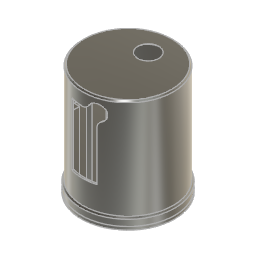
meshtastic-heltec-holder v7 (Autodesk Fusion 360 design; units mm, degrees)
Autodesk Fusion 360 part; units mm, degrees
note: some values were not read from the file. Set by a fixed rule: which sketch regions a step uses.
sketch "boden" plane through (0, 0, 0) normal (0, 0, 1) x (1, 0, 0)
  circle A0 centre (0, 0) radius 30
  line L0 (-11, -23) -> (11, -23)
  line L1 (11, -23) -> (11, -15)
  line L2 (11, -15) -> (-11, -15)
  line L3 (-11, -15) -> (-11, -23)
  line L4 (-11, -23) -> (-8, -23)
  line L5 (-8, -23) -> (-8, -25)
  line L6 (-8, -25) -> (-11, -25)
  line L7 (-11, -25) -> (-11, -23)
  line L8 (11, -23) -> (8, -23)
  line L9 (8, -23) -> (8, -25)
  line L10 (8, -25) -> (11, -25)
  line L11 (11, -25) -> (11, -23)
  line L12 (-11, -15) -> (-8, -15)
  line L13 (-8, -15) -> (-8, -13)
  line L14 (-8, -13) -> (-11, -13)
  line L15 (-11, -13) -> (-11, -15)
  line L16 (11, -15) -> (8, -15)
  line L17 (8, -15) -> (8, -13)
  line L18 (8, -13) -> (11, -13)
  line L19 (11, -13) -> (11, -15)
  line L20 (11, -13) -> (13, -13)
  line L21 (13, -13) -> (13, -25)
  line L22 (13, -25) -> (11, -25)
  line L23 (11, -25) -> (11, -13)
  line L24 (-11, -25) -> (-13, -25)
  line L25 (-13, -25) -> (-13, -13)
  line L26 (-13, -13) -> (-11, -13)
  line L27 (-11, -13) -> (-11, -25)
  line L28 (8, -15) -> (-8, -15)
  line L29 (-8, -15) -> (-8, -6)
  line L30 (-8, -6) -> (8, -6)
  line L31 (8, -6) -> (8, -15)
  line L32 (-13, -13) -> (-11, -13)
  line L33 (-11, -13) -> (-11, -4)
  line L34 (-11, -4) -> (-13, -4)
  line L35 (-13, -4) -> (-13, -13)
  line L36 (13, -4) -> (13, -6)
  line L37 (13, -6) -> (-11, -6)
  line L38 (-11, -6) -> (-11, -4)
  line L39 (11, -13) -> (13, -13)
  line L40 (13, -13) -> (13, -6)
  line L41 (13, -6) -> (11, -6)
  line L42 (11, -6) -> (11, -13)
  line L43 (13, -4) -> (3, -4)
  line L44 (3, -4) -> (3, -6)
  line L45 (3, -6) -> (13, -6)
  line L46 (13, -6) -> (13, -4)
  line L47 (-11, -4) -> (-3, -4)
  line L48 (-3, -4) -> (-3, -6)
  line L49 (-3, -6) -> (-11, -6)
  line L50 (-11, -6) -> (-11, -4)
  line L51 (-26.5, -4) -> (26.5, -4)
  line L52 (26.5, -4) -> (26.5, 2)
  line L53 (26.5, 2) -> (-26.5, 2)
  line L54 (-26.5, 2) -> (-26.5, -4)
  line L55 (-13, -5) -> (-13, -4)
  line L56 (-13, -4) -> (-27.5, -4)
  line L57 (-27.5, -4) -> (-27.5, -5)
  line L58 (-27.5, -5) -> (-13, -5)
  line L59 (-13, -5) -> (-13, -4)
  line L60 (-26.5, -4) -> (-27.5, -4)
  line L61 (-27.5, -4) -> (-27.5, 3)
  line L62 (-27.5, 3) -> (-26.5, 3)
  line L63 (-26.5, 3) -> (-26.5, -4)
  line L64 (-26.5, 3) -> (27.5, 3)
  line L65 (27.5, 3) -> (27.5, 2)
  line L66 (27.5, 2) -> (-26.5, 2)
  line L67 (-26.5, 2) -> (-26.5, 3)
  line L68 (27.5, 2) -> (26.5, 2)
  line L69 (26.5, 2) -> (26.5, -5)
  line L70 (26.5, -5) -> (27.5, -5)
  line L71 (27.5, -5) -> (27.5, 2)
  line L72 (26.5, -5) -> (13, -5)
  line L73 (13, -5) -> (13, -4)
  line L74 (13, -4) -> (26.5, -4)
  line L75 (26.5, -4) -> (26.5, -5)
  line L76 (2, 2) -> (-2, 2)
  line L77 (-2, 2) -> (-2, 3)
  line L78 (-2, 3) -> (2, 3)
  line L79 (2, 3) -> (2, 2)
  line L80 (10, 3) -> (-10, 3)
  line L81 (-10, 3) -> (-10, 17)
  line L82 (-10, 17) -> (10, 17)
  line L83 (10, 17) -> (10, 3)
  line L84 (8, 17) -> (-8, 17)
  line L85 (-8, 17) -> (-8, 5)
  line L86 (-8, 5) -> (8, 5)
  line L87 (8, 5) -> (8, 17)
  line L88 (2, 3) -> (-2, 3)
  line L89 (-2, 5) -> (2, 5)
  line L90 (1, 3) -> (-1, 3)
  line L91 (-1, 3) -> (-1, 5)
  line L92 (-1, 5) -> (1, 5)
  line L93 (1, 5) -> (1, 3)
  line L94 (1, 5) -> (-1, 5)
  line L95 (-1, 5) -> (-1, 13)
  line L96 (-1, 13) -> (1, 13)
  line L97 (1, 13) -> (1, 5)
  circle A1 centre (0, 13) radius 3.1
  circle A2 centre (0, 0) radius 28
  circle A3 centre (0, 0) radius 29
  line L98 (-27.8388, 3) -> (-27.5, 3)
  line L99 (-25.5, 3) -> (-25.5, 7.5)
  line L100 (-25.5, 7.5) -> (-26.9768, 7.5)
  line L101 (27.5, 3) -> (27.8388, 3)
  line L102 (0, 0) -> (0, 40) construction
  line L103 (25.5, 3) -> (25.5, 7.5)
  line L104 (25.5, 7.5) -> (26.9768, 7.5)
  line L105 (-5, 5) -> (5, 5)
  line L106 (5, 5) -> (5, 2)
  line L107 (5, 2) -> (-5, 2)
  line L108 (-5, 2) -> (-5, 5)
  line L109 (27.5, -5) -> (27.55, -5)
  line L110 (-27.5, -4) -> (-27.7128, -4)
  line L111 (-8, -25) -> (-8, -26.8328)
  line L112 (8, -25) -> (8, -26.8328)
  circle A4 centre (0, 13) radius 6.75
  dimension "d1" = 60
  dimension "d4" = 22
  dimension "d5" = 8
  dimension "d6" = 11
  dimension "d7" = 15
  dimension "d8" = 53
  dimension "d9" = 6
  dimension "d10" = 1
  dimension "d11" = 26.5
  dimension "d18" = 6.2
  dimension "d23" = 58
  dimension "d24" = 40
  dimension "d37" = 13.5
  constraint coincident A0.centre A2.centre
  constraint horizontal L0
  constraint vertical L1
  constraint horizontal L2
  constraint vertical L3
  constraint horizontal L4
  constraint vertical L5
  constraint horizontal L6
  constraint vertical L7
  constraint horizontal L8
  constraint vertical L9
  constraint horizontal L10
  constraint vertical L11
  constraint horizontal L12
  constraint vertical L13
  constraint horizontal L14
  constraint vertical L15
  constraint horizontal L16
  constraint vertical L17
  constraint horizontal L18
  constraint vertical L19
  constraint horizontal L20
  constraint vertical L21
  constraint horizontal L22
  constraint vertical L23
  constraint horizontal L24
  constraint vertical L25
  constraint horizontal L26
  constraint vertical L27
  constraint horizontal L28
  constraint vertical L29
  constraint horizontal L30
  constraint vertical L31
  constraint horizontal L32
  constraint vertical L33
  constraint horizontal L34
  constraint vertical L35
  constraint vertical L36
  constraint horizontal L37
  constraint vertical L38
  constraint horizontal L39
  constraint vertical L40
  constraint horizontal L41
  constraint vertical L42
  constraint horizontal L43
  constraint vertical L44
  constraint horizontal L45
  constraint vertical L46
  constraint coincident L30 L44.end
  constraint coincident L37 L44.end
  constraint horizontal L47
  constraint vertical L48
  constraint horizontal L49
  constraint vertical L50
  constraint coincident L30 L48.end
  constraint horizontal L51
  constraint vertical L52
  constraint horizontal L53
  constraint vertical L54
  constraint vertical L55
  constraint horizontal L56
  constraint vertical L57
  constraint horizontal L58
  constraint vertical L59
  constraint horizontal L60
  constraint vertical L61
  constraint horizontal L62
  constraint vertical L63
  constraint horizontal L64
  constraint vertical L65
  constraint horizontal L66
  constraint vertical L67
  constraint horizontal L68
  constraint vertical L69
  constraint horizontal L70
  constraint vertical L71
  constraint horizontal L72
  constraint vertical L73
  constraint horizontal L74
  constraint vertical L75
  constraint horizontal L76
  constraint vertical L77
  constraint horizontal L78
  constraint vertical L79
  constraint coincident L64 L77.end
  constraint horizontal L80
  constraint vertical L81
  constraint horizontal L82
  constraint vertical L83
  constraint coincident L64 L80.start
  constraint horizontal L84
  constraint vertical L85
  constraint horizontal L86
  constraint vertical L87
  constraint coincident L82 L84.start
  constraint horizontal L88
  constraint horizontal L89
  constraint coincident L86 L89.start
  constraint horizontal L90
  constraint vertical L91
  constraint horizontal L92
  constraint vertical L93
  constraint coincident L89 L91.end
  constraint coincident L80 L90.start
  constraint horizontal L94
  constraint vertical L95
  constraint horizontal L96
  constraint vertical L97
  constraint midpoint L96 A1.centre
  constraint coincident A2 L98.start
  constraint perpendicular L61 L98
  constraint coincident L64 L99.start
  constraint perpendicular L64 L99
  constraint coincident A2 L100.end
  constraint perpendicular L99 L100
  constraint coincident A2 L101.end
  constraint perpendicular L65 L101
  constraint vertical L102
  constraint symmetric L99.start L102 L103.start
  constraint symmetric L99.end L102 L103.end
  constraint symmetric L100.end L102 L104.end
  constraint horizontal L105
  constraint vertical L106
  constraint horizontal L107
  constraint vertical L108
  constraint coincident L53 L106.end
  constraint coincident L86 L105.start
  constraint coincident A2 L109.end
  constraint perpendicular L71 L109
  constraint coincident A2 L110.end
  constraint perpendicular L57 L110
  constraint coincident A2 L111.end
  constraint perpendicular L6 L111
  constraint coincident A2 L112.end
  constraint perpendicular L10 L112
  constraint concentric A1 A4
  measures "d1" diameter of A0
  measures "d4" distance of L0.start L0.end
  measures "d5" distance of L0.start L2.end
  measures "d6" distance of A0.centre L1
  measures "d7" distance of A0.centre L28
  measures "d8" distance of L51.start L51.end
  measures "d9" distance of L51.start L53.end
  measures "d10" distance of L54 L57
  measures "d11" distance of A0.centre L54
  measures "d18" diameter of A1
  measures "d23" diameter of A3
  measures "d24" distance of A0.centre L102.end
  measures "d37" diameter of A4
extrude "Extrude1" add sketch "boden" against normal blind 2 contours A0 | L0 L1 L2 L3 L4 L8 L12 L16 L23 L27 L28 | L3 L7 L15 L24 L25 L26 L27 L32 A2 | L0 L4 L5 L6 L7 L27 | L0 L5 L9 A2 L111 L112 | L2 L12 L13 L14 L15 L27 L29 | L6 L24 A2 L111 | L0 L8 L9 L10 L11 L23 | L2 L13 L17 L28 L29 L30 L31 L37 L45 L49 | L14 L29 L33 L37 L49 | L26 L32 L33 L34 L35 L38 L50 L51 L55 L59 | L24 L25 A2 | L1 L11 L19 L20 L21 L22 L23 L39 A2 | L10 L22 A2 L112 | L2 L16 L17 L18 L19 L23 L31 | L25 L35 L57 L58 A2 L110 | L30 L33 L37 L38 L47 L48 L49 L50 L51 | L18 L31 L37 L42 L45 | L35 L51 L55 L56 L57 L58 L59 L60 | L34 L43 L47 L51 L52 L53 L54 L56 L63 L66 L69 L74 L76 L107 | L61 A2 L98 L110 | L20 L37 L39 L40 L41 L42 L45 | L21 L22 A2 | L30 L36 L37 L41 L43 L44 L45 L46 L51 L73 | L30 L37 L44 L48 L51 | L62 L64 A2 L98 L99 L100 | L54 L56 L60 L61 L62 L63 L67 | L21 L36 L40 L46 L70 L72 A2 L109 | L64 L81 L82 L83 L84 A2 L99 L100 L103 L104 A4 | L65 L71 A2 L101 L109 | L53 L63 L64 L66 L67 L80 L108 | L36 L46 L51 L69 L72 L73 L74 L75 | L64 A2 L101 L103 L104 | L52 L66 L68 L69 L70 L71 L75 | L53 L64 L66 L77 L80 L107 L108 | L53 L64 L65 L66 L68 L80 L106 | L53 L64 L66 L76 L77 L78 L79 L80 L88 L90 L107 | L64 L78 L80 L86 L88 L89 L91 L105 L108 | L64 L80 L81 L82 L85 L86 L108 | L53 L64 L66 L79 L80 L106 L107 | L82 L84 L85 L86 L89 L95 L105 A4 | L64 L80 L82 L83 L86 L87 L106 | L64 L78 L80 L86 L88 L89 L93 L105 L106 | L64 L78 L80 L86 L88 L89 L90 L91 L92 L93 L94 L105 | L86 L89 L92 L94 L95 L97 L105 A4 | L82 L84 L86 L87 L89 L97 L105 A4 | L82 L84 A4 | L82 L84 L95 L97 A1 A4 | L95 L97 A1 A4 | L95 L96 L97 A1 | L95 L96 L97 A1 | A3 makes body 1
extrude "Extrude2" add sketch "boden" along normal blind 48 contours L3 L7 L15 L24 L25 L26 L27 L32 A2 | L0 L4 L5 L6 L7 L27 | L2 L12 L13 L14 L15 L27 L29 | L0 L8 L9 L10 L11 L23 | L14 L29 L33 L37 L49 | L26 L32 L33 L34 L35 L38 L50 L51 L55 L59 | L24 L25 A2 | L1 L11 L19 L20 L21 L22 L23 L39 A2 | L2 L16 L17 L18 L19 L23 L31 | L30 L33 L37 L38 L47 L48 L49 L50 L51 | L18 L31 L37 L42 L45 | L20 L37 L39 L40 L41 L42 L45 | L21 L22 A2 | L30 L36 L37 L41 L43 L44 L45 L46 L51 L73 bodies 1
extrude "Extrude3" add sketch "boden" along normal blind 60 contours L35 L51 L55 L56 L57 L58 L59 L60 | L54 L56 L60 L61 L62 L63 L67 | L53 L63 L64 L66 L67 L80 L108 | L36 L46 L51 L69 L72 L73 L74 L75 | L52 L66 L68 L69 L70 L71 L75 | L53 L64 L66 L77 L80 L107 L108 | L53 L64 L65 L66 L68 L80 L106 | L53 L64 L66 L76 L77 L78 L79 L80 L88 L90 L107 | L53 L64 L66 L79 L80 L106 L107 bodies 1
extrude "Extrude4" cut sketch "boden" along normal blind 76 contours L53 L64 L66 L76 L77 L78 L79 L80 L88 L90 L107 bodies 1
extrude "Extrude5" add sketch "boden" along normal blind 20 contours L64 L78 L80 L86 L88 L89 L91 L105 L108 | L64 L80 L81 L82 L85 L86 L108 | L82 L84 L85 L86 L89 L95 L105 A4 | L64 L80 L82 L83 L86 L87 L106 | L64 L78 L80 L86 L88 L89 L93 L105 L106 | L82 L84 L86 L87 L89 L97 L105 A4 | L82 L84 L95 L97 A1 A4 bodies 1
extrude "Extrude6" cut sketch "boden" along normal blind 17 contours L82 L84 L85 L86 L89 L95 L105 A4 | L82 L84 L86 L87 L89 L97 L105 A4 | L82 L84 L95 L97 A1 A4 bodies 1
extrude "Extrude7" add sketch "boden" along normal blind 3 contours A3 bodies 1
extrude "Extrude8" add sketch "boden" along normal blind 6 contours L62 L64 A2 L98 L99 L100 | L64 A2 L101 L103 L104 bodies 1
move_face "OffsetFaces1" offset -0.5 1 faces at (-11, -17.6667, 16) on bodies 1
move_face "OffsetFaces2" offset -0.5 1 faces at (11, -20.3333, 16) on bodies 1
extrude "Extrude9" cut sketch "boden" along normal blind 5 contours L53 L64 L66 L77 L80 L107 L108 | L53 L64 L66 L76 L77 L78 L79 L80 L88 L90 L107 | L64 L78 L80 L86 L88 L89 L91 L105 L108 | L53 L64 L66 L79 L80 L106 L107 | L64 L78 L80 L86 L88 L89 L93 L105 L106 | L64 L78 L80 L86 L88 L89 L90 L91 L92 L93 L94 L105 bodies 1
extrude "Extrude10" add 2 faces at (10.8333, -8.6667, 48) (-10.8333, -8.6667, 48) along direction (0, 0, 1) blind 5 on bodies 1 bodies 1
sketch "window cutout" plane through (0, -15, 0) normal (0, -1, 0) x (1, 0, 0)
  line L0 (8, 0) -> (11.5, 0)
  line L1 (11.5, 0) -> (11.5, 53)
  line L2 (11.5, 53) -> (8, 53)
  line L3 (8, 53) -> (8, 0)
  line L4 (-8, 20) -> (8, 20)
  line L5 (8, 20) -> (8, 60)
  line L6 (8, 60) -> (-8, 60)
  line L7 (-8, 60) -> (-8, 20)
  circle A0 centre (8, 60) radius 5
  dimension "d35" = 40
  dimension "d36" = 20
  dimension "d50" = 10
  constraint horizontal L4
  constraint vertical L5
  constraint horizontal L6
  constraint vertical L7
  constraint coincident L5.end L6.start
  measures "d35" distance of L4.start L6.end
  measures "d36" distance of origin L4
  measures "d50" diameter of A0
extrude "Extrude11" add sketch "boden" along normal blind 53 contours L6 L24 A2 L111 | L10 L22 A2 L112 bodies 1
extrude "Extrude12" add sketch "boden" along normal blind 60 contours L61 A2 L98 L110 | L65 L71 A2 L101 L109 bodies 1
extrude "Extrude13" add 1 faces at (2.0698, -28.2085, 3) along direction (0, 0, 1) blind 65 separate body on bodies 1 makes body 2
sketch "shell_ceiling" plane through (0, 0, 68) normal (0, 0, 1) x (-1, 0, 0)
  line L0 (-13, 24.7992) -> (-13, 25)
  line L1 (-13, 25) -> (-12.6095, 25)
  arc A0 (12.6095, 25) -> (-12.6095, 25) centre (0, 0) ccw
  line L2 (12.6095, 25) -> (13, 25)
  line L3 (13, 25) -> (13, 24.7992)
  arc A1 (-13, 24.7992) -> (13, 24.7992) centre (0, 0) ccw
  circle A2 centre (0, 0) radius 29
extrude "Extrude14" add sketch "shell_ceiling" along normal blind 1 contours L0 L1 A0 L2 L3 A1 | A2 bodies 2
extrude "Extrude15" cut sketch "boden" along normal blind 80 contours L82 L84 A4 | L82 L84 L95 L97 A1 A4 | L95 L97 A1 A4 | L95 L96 L97 A1 | L95 L96 L97 A1 bodies 2
extrude "Extrude16" cut sketch "window cutout" along normal blind 30 contours L3 L4 L5 L6 L7 A0 | L5 L6 A0 picked at (4.6836, 59.7628) bodies 2
extrude "Extrude17" cut sketch "window cutout" along normal blind 20 contours L5 L6 A0 picked at (5.4012, 62.0725) bodies 2
fillet "Fillet1" radius 4 2 edges at (3, -28.3416, 60) (8, -27.3538, 55) on bodies 2
extrude "Extrude18" add 1 faces at (29.447, -2.9312, 0) along direction (0, 0, 1) blind 5 separate body on bodies 1 makes body 3
combine "Combine1" operation add target body 3 tool bodies 2
chamfer "Chamfer1" distance 1 angle 45 1 edges at (-27.9698, -10.8485, 5) on bodies 3
move_face "OffsetFaces3" offset -0.1 1 faces at (28.8559, -2.8875, 1) on bodies 3
chamfer "Chamfer2" distance 1 angle 45 1 edges at (27.0375, 10.4868, 69) on bodies 3
chamfer "Chamfer3" distance 1 angle 45 1 edges at (-6.2932, 10.5591, 68) on bodies 3
equation "d11 = ( 53 / 2 ) * 1 mm"
named bodies: "decorative_shell", "shell"
